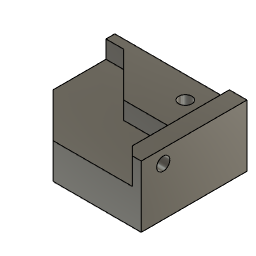
f1 (Autodesk Fusion 360 design; units mm, degrees)
Autodesk Fusion 360 part; units mm, degrees
sketch "Sketch1" plane through (0, 0, 0) normal (0, 0, 1) x (1, 0, 0)
  line L0 (50, 0) -> (150, 0)
  line L1 (150, 0) -> (150, 120)
  line L2 (150, 120) -> (0, 120)
  line L3 (0, 120) -> (0, 50)
  line L4 (0, 50) -> (50, 0)
  line L5 (0, 50) -> (0, 0)
  line L6 (0, 0) -> (50, 0)
  line L7 (0, 110) -> (20, 110)
  line L8 (20, 110) -> (70, 60)
  line L9 (70, 60) -> (130, 60)
  line L10 (130, 60) -> (130, 120)
  line L11 (130, 60) -> (130, 10)
  line L12 (130, 10) -> (140, 0)
  dimension "d2" = 120
  dimension "d3" = 50
  dimension "d4" = 135
  dimension "d5" = 10
  dimension "d6" = 10
  dimension "d7" = 10
  dimension "d8" = 60
  dimension "d9" = 135
  dimension "d10" = 20
  dimension "d17" = 60
  constraint horizontal L0
  constraint vertical L1
  constraint horizontal L2
  constraint vertical L3
  constraint coincident L5.end L6.start
  constraint vertical L5
  constraint horizontal L6
  constraint equal L5 L6
  constraint coincident L3 L7.start
  constraint perpendicular L3 L7
  constraint perpendicular L3 L9
  constraint coincident L2 L10.end
  constraint perpendicular L2 L10
  constraint perpendicular L9 L11
  constraint coincident L0 L12.end
  measures "d2" distance of L5.end L2.end
  measures "d3" distance of L5.end L0.start
  measures "d4" angle of L0 L12
  measures "d5" distance of L0 L11.end
  measures "d6" distance of L2 L7
  measures "d7" distance of L0.end L12.end
  measures "d8" distance of L2 L9
  measures "d9" angle of L8 L9
  measures "d10" distance of L7.start L7.end
  measures "d17" distance of L8.end L9.end
extrude "Extrude1" add sketch "Sketch1" along normal blind 40 contours L0 L3 L4 L7 L8 L9 L11 L12
extrude "Extrude2" add sketch "Sketch1" along normal blind 60 contours L2 L3 L7 L8 L9 L10
extrude "Extrude3" add sketch "Sketch1" along normal blind 70 contours L0 L1 L2 L10 L11 L12
sketch "Sketch2" plane through (0, 0, 60) normal (0, 0, 1) x (-1, 0, 0)
  line L0 (-130, -60) -> (-130, -120)
  line L1 (-130, -120) -> (0, -120)
  line L2 (0, -120) -> (0, -110)
  line L3 (0, -110) -> (-20, -110)
  line L4 (-20, -110) -> (-70, -60)
  line L5 (-70, -60) -> (-130, -60)
  circle A0 centre (-105, -95) radius 7.5
  dimension "d23" = 15
  dimension "d24" = 25
  dimension "d25" = 25
  measures "d23" diameter of A0
  measures "d24" distance of L0 A0.centre
  measures "d25" distance of L1 A0.centre
sketch "Sketch3" plane through (130, 0, 0) normal (-1, 0, 0) x (0, -1, 0)
  line L0 (-60, 40) -> (-10, 40)
  line L1 (-10, 40) -> (-10, 70)
  line L2 (-10, 70) -> (-120, 70)
  line L3 (-60, 60) -> (-60, 40)
  circle A0 centre (-25, 55) radius 7.5
  line L4 (-120, 70) -> (-120, 60)
  line L5 (-120, 60) -> (-60, 60)
  dimension "d26" = 15
  dimension "d27" = 15
  dimension "d28" = 15
  measures "d26" diameter of A0
  measures "d27" distance of L2 A0.centre
  measures "d28" distance of L1 A0.centre
extrude "Extrude4" cut sketch "Sketch3" against normal blind 30 contours A0
extrude "Extrude5" cut sketch "Sketch2" against normal blind 50 contours A0
